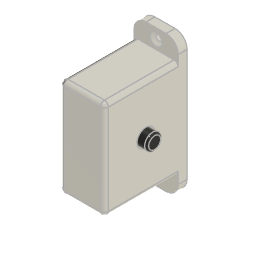
Exit Button Holder v2 (Autodesk Fusion 360 design; units mm, degrees)
Autodesk Fusion 360 part; units mm, degrees
note: some values were not read from the file. Set by a fixed rule: which sketch regions a step uses.
sketch "Sketch2" plane through (0, 0, 0) normal (1, 0, 0) x (0, 1, 0) in component "Switch PCB"
  line L0 (-3, 0) -> (-26, 0)
  line L1 (-29, 3) -> (-29, 33.5)
  line L2 (-26, 36.5) -> (-3, 36.5)
  line L3 (0, 33.5) -> (0, 3)
  line L4 (-14.5, 0) -> (-14.5, 3) construction
  line L5 (0, 18.25) -> (-3, 18.25) construction
  line L6 (-3, 33.5) -> (-26, 33.5) construction
  line L7 (-26, 33.5) -> (-26, 3) construction
  line L8 (-26, 3) -> (-3, 3) construction
  line L9 (-3, 3) -> (-3, 33.5) construction
  circle A0 centre (-26, 33.5) radius 1.5
  circle A1 centre (-3, 33.5) radius 1.5
  circle A2 centre (-26, 3) radius 1.5
  circle A3 centre (-3, 3) radius 1.5
  arc A4 (-26, 36.5) -> (-29, 33.5) centre (-26, 33.5) ccw
  arc A5 (0, 33.5) -> (-3, 36.5) centre (-3, 33.5) ccw
  arc A6 (-29, 3) -> (-26, 0) centre (-26, 3) ccw
  arc A7 (-3, 0) -> (0, 3) centre (-3, 3) ccw
  line L10 (-8.65, 7.5) -> (-20.35, 7.5)
  line L11 (-20.35, 7.5) -> (-20.35, 0)
  line L12 (-20.35, 0) -> (-8.65, 0)
  line L13 (-8.65, 0) -> (-8.65, 7.5)
  line L14 (-14.5, 0) -> (-14.5, 18.25) construction
  line L15 (-14.5, 18.25) -> (0, 18.25) construction
  circle A8 centre (-14.5, 18.25) radius 4
  circle A9 centre (-14.5, 18.25) radius 5.5
  line L16 (-6.15, 7.5) -> (-22.85, 7.5)
  line L17 (-22.85, 7.5) -> (-22.85, 0)
  line L18 (-22.85, 0) -> (-6.15, 0)
  line L19 (-6.15, 0) -> (-6.15, 7.5)
  point P0 (-29, 0)
  point P1 (0, 36.5)
  point P2 (-14.5, 3)
  point P3 (-3, 18.25)
  point P4 (-14.5, 0)
  point P5 (-14.5, -4)
  point P6 (-14.5, 0)
  dimension "d11" = 29
  dimension "d12" = 36.5
  dimension "d13" = 3
  dimension "d14" = 3
  dimension "d15" = 3
  dimension "d16" = 3
  dimension "d17" = 3
  dimension "d18" = 3
  dimension "d19" = 3
  dimension "d20" = 3
  dimension "d21" = 3
  dimension "d22" = 3
  dimension "d23" = 23
  dimension "d24" = 30.5
  dimension "d25" = 11.7
  dimension "d26" = 7.5
  dimension "d27" = 4
  dimension "d164" = 8
  dimension "d165" = 11
  dimension "d175" = 16.7
  dimension "d176" = 7.5
  constraint horizontal L0
  constraint vertical L1
  constraint horizontal L2
  constraint vertical L3
  constraint perpendicular L0 L4
  constraint perpendicular L3 L5
  constraint horizontal L6
  constraint vertical L7
  constraint horizontal L8
  constraint vertical L9
  constraint midpoint L8 P2
  constraint coincident P2 L4.end
  constraint midpoint L9 P3
  constraint coincident P3 L5.end
  constraint coincident L6.end L7.start
  constraint coincident L6.start L9.end
  constraint coincident L7.end L8.start
  constraint coincident L8.end L9.start
  constraint tangent L1 A4
  constraint tangent L2 A4
  constraint coincident L3 L5.start
  constraint coincident P1 L2
  constraint coincident P1 L3
  constraint tangent L2 A5
  constraint tangent L3 A5
  constraint coincident L0 P6
  constraint coincident P0 L1
  constraint coincident P0 L0
  constraint tangent L1 A6
  constraint tangent L0 A6
  constraint coincident origin L3
  constraint coincident origin L0
  constraint tangent L3 A7
  constraint tangent L0 A7
  constraint horizontal L10
  constraint vertical L11
  constraint horizontal L12
  constraint vertical L13
  constraint midpoint L12 P6
  constraint coincident P6 L4.start
  constraint coincident P6 P4
  constraint vertical L14
  constraint horizontal L15
  constraint coincident L14.end L15.start
  constraint horizontal L16
  constraint vertical L17
  constraint horizontal L18
  constraint vertical L19
  constraint midpoint L18 P6
  measures "d11" distance of origin P0
  measures "d12" distance of origin P1
  measures "d13" distance of P6 P2
  measures "d14" distance of L5.start P3
  measures "d15" diameter of A0
  measures "d16" diameter of A1
  measures "d17" diameter of A2
  measures "d18" diameter of A3
  measures "d19" radius of A4
  measures "d20" radius of A5
  measures "d21" radius of A6
  measures "d22" radius of A7
  measures "d23" distance of L7.end L8.end
  measures "d24" distance of L6.end L7.end
  measures "d25" distance of L10.start L10.end
  measures "d26" distance of L10.start L12.end
  measures "d27" distance of P6 P5
  measures "d164" diameter of A8
  measures "d165" diameter of A9
  measures "d175" distance of L16.start L16.end
  measures "d176" distance of L16.start L18.end
extrude "Extrude1" add sketch "Sketch2" against normal blind 1.6 contours L0 L1 L2 L3 A4 A5 A6 A7 L10 L16 L17 L19 | L0 L13 L16 L18 L19 | L0 L10 L11 L12 L13 L16 L18 | L0 L11 L16 L17 L18 | A8 | A9 makes body 1 in component "Switch PCB"
extrude "Extrude2" add sketch "Sketch2" along normal blind 5 contours L0 L10 L11 L12 L13 L16 L18 bodies 1 in component "Switch PCB"
extrude "Extrude3" add sketch "Sketch2" against normal blind 5 from surface at -1.6 contours L0 L13 L16 L18 L19 | L0 L10 L11 L12 L13 L16 L18 | L0 L11 L16 L17 L18 bodies 1 in component "Switch PCB"
sketch "Sketch1" plane through (0, 0, 0) normal (0, 1, 0) x (1, 0, 0) in component "PIR Holder"
  line L0 (0, 0) -> (0, -5) construction
  circle A0 centre (0, -5) radius 1.5
  line L1 (-11, -68) -> (11, -68)
  line L2 (11, -68) -> (11, 0)
  line L3 (11, 0) -> (-11, 0)
  line L4 (-11, 0) -> (-11, -68)
  line L5 (0, -68) -> (0, -63) construction
  circle A1 centre (0, -63) radius 1.5
  dimension "d1" = 5
  dimension "d2" = 3
  dimension "d3" = 22
  dimension "d4" = 68
  dimension "d5" = 5
  dimension "d6" = 3
  constraint coincident L0.start origin
  constraint vertical L0
  constraint coincident L0.end A0.centre
  constraint horizontal L1
  constraint vertical L2
  constraint horizontal L3
  constraint vertical L4
  constraint midpoint L3 L0.start
  constraint midpoint L1 L5.start
  constraint perpendicular L1 L5
  constraint coincident L5.end A1.centre
  measures "d1" distance of L0.start L0.end
  measures "d2" diameter of A0
  measures "d3" distance of L1.start L1.end
  measures "d4" distance of L1.start L3.end
  measures "d5" distance of L5.start L5.end
  measures "d6" diameter of A1
extrude "Extrude1'" add sketch "Sketch1" against normal blind 4.5 separate body makes body 2 in component "PIR Holder"
fillet "Fillet1" radius 6 4 edges at (11, -2.25, 68) (-11, -2.25, 68) (11, -2.25, 0) (-11, -2.25, 0) on bodies 2 in component "PIR Holder"
sketch "Sketch2 (2)" plane through (-11, 0, 0) normal (-1, 0, 0) x (0, -1, 0) in component "PIR Holder"
  line L0 (0, 6) -> (4.5, 6)
  line L1 (4.5, 6) -> (4.5, 62)
  line L2 (4.5, 62) -> (0, 62)
  line L3 (0, 62) -> (0, 6)
  line L4 (4.5, 62) -> (4.5, 6)
  line L5 (0, 0) -> (0, 15) construction
  line L6 (0, 15) -> (9, 15) construction
  dimension "d64" = 15
  dimension "d65" = 9
  constraint coincident L5.start origin
  constraint parallel L3 L5
  constraint perpendicular L4 L6
  measures "d64" distance of L5.start L5.end
  measures "d65" distance of L5.end L6.end
sketch "Sketch3" plane through (0, 0, 0) normal (1, 0, 0) x (0, 1, 0) in component "PIR Holder"
  line L0 (-32, 52.5) -> (-9, 52.5)
sketch "Sketch4" plane through (11, 0, 0) normal (1, 0, 0) x (0, 1, 0) in component "PIR Holder"
  line L0 (-4.5, 6) -> (0, 6)
  line L1 (0, 6) -> (0, 62)
  line L2 (0, 62) -> (-4.5, 62)
  line L3 (-4.5, 62) -> (-4.5, 6)
  line L4 (-26.35, 16) -> (-26.35, 23.5)
  line L5 (-26.35, 23.5) -> (-14.65, 23.5)
  line L6 (-14.65, 23.5) -> (-14.65, 16)
  line L7 (-14.65, 16) -> (-9, 16)
  arc A0 (-9, 16) -> (-6, 19) centre (-9, 19) ccw
  line L8 (-6, 19) -> (-6, 49.5)
  arc A1 (-6, 49.5) -> (-9, 52.5) centre (-9, 49.5) ccw
  line L9 (-9, 52.5) -> (-32, 52.5)
  arc A2 (-32, 52.5) -> (-35, 49.5) centre (-32, 49.5) ccw
  line L10 (-35, 49.5) -> (-35, 19)
  arc A3 (-35, 19) -> (-32, 16) centre (-32, 19) ccw
  line L11 (-32, 16) -> (-26.35, 16)
  circle A4 centre (-32, 19) radius 1.5
  circle A5 centre (-9, 49.5) radius 1.5
  circle A6 centre (-9, 19) radius 1.5
  circle A7 centre (-32, 49.5) radius 1.5
  line L12 (-14.65, 16) -> (-14.65, 23.5)
  line L13 (-14.65, 23.5) -> (-26.35, 23.5)
  line L14 (-26.35, 23.5) -> (-26.35, 16)
  line L15 (-26.35, 16) -> (-14.65, 16)
  line L16 (-20.5, 52.5) -> (-20.5, 56.5) construction
  line L17 (-20.5, 56.5) -> (-4.5, 56.5)
  line L18 (-4.5, 56.5) -> (-4.5, 12)
  line L19 (-20.5, 56.5) -> (-32, 56.5)
  line L20 (-32, 56.5) -> (-39, 56.5)
  line L21 (-39, 56.5) -> (-39, 12)
  line L22 (-39, 12) -> (-4.5, 12)
  circle A8 centre (-32, 49.5) radius 3
  circle A9 centre (-9, 49.5) radius 3
  circle A10 centre (-32, 19) radius 3
  circle A11 centre (-9, 19) radius 3
  circle A12 centre (-32, 49.5) radius 1
  circle A13 centre (-9, 49.5) radius 1
  circle A14 centre (-32, 19) radius 1
  circle A15 centre (-9, 19) radius 1
  line L23 (-35, 34.25) -> (-39, 34.25) construction
  line L24 (-32, 52.5) -> (-32, 56.5) construction
  line L25 (-20.5, 16) -> (-20.5, 12) construction
  circle A16 centre (-20.5, 34.25) radius 4
  circle A17 centre (-20.5, 34.25) radius 4.5
  point P0 (-20.5, 52.5)
  dimension "d82" = 4
  dimension "d89" = 6
  dimension "d90" = 6
  dimension "d91" = 6
  dimension "d92" = 6
  dimension "d93" = 2
  dimension "d94" = 2
  dimension "d95" = 2
  dimension "d96" = 2
  dimension "d163" = 4
  dimension "d178" = 4
  dimension "d179" = 0.5
  constraint coincident L3 L18.end
  constraint coincident L3 L17.end
  constraint perpendicular L3 L17
  constraint perpendicular L16 L19
  constraint perpendicular L16 L20
  constraint concentric A2 A8
  constraint concentric A1 A9
  constraint concentric A3 A10
  constraint concentric A0 A11
  constraint concentric A8 A12
  constraint concentric A9 A13
  constraint concentric A10 A14
  constraint concentric A11 A15
  constraint vertical L16
  constraint midpoint L9 P0
  constraint coincident P0 L16.start
  constraint midpoint L10 L23.start
  constraint midpoint L21 L23.end
  constraint coincident L9.end A2.start
  constraint vertical L24
  constraint vertical L21
  constraint horizontal L22
  constraint midpoint L15 L25.start
  constraint coincident L22 L25.end
  constraint perpendicular L22 L25
  constraint coincident L18 L22.end
  constraint coincident L18.end L22.end
  measures "d82" distance of P0 L16.end
  measures "d89" diameter of A8
  measures "d90" diameter of A9
  measures "d91" diameter of A10
  measures "d92" diameter of A11
  measures "d93" diameter of A12
  measures "d94" diameter of A13
  measures "d95" diameter of A14
  measures "d96" diameter of A15
  measures "d163" distance of L23.start L23.end
  measures "d178" distance of L25.start L25.end
extrude "Extrude5" add sketch "Sketch2" along normal blind 7.3 contours A8 | A9 bodies 1 in component "Switch PCB"
extrude "Extrude6" add sketch "Sketch2" along normal blind 6.8 from surface at 7.3 contours A8 bodies 1 in component "Switch PCB"
fillet "Fillet1'" radius 1 1 edges at (14.1, -18.2293, 16.8035) on bodies 1 in component "Switch PCB"
fillet "Fillet2" radius 1 1 edges at (7.3, -19.6278, 16.2611) on bodies 1 in component "Switch PCB"
chamfer "Chamfer1" distance 1 angle 45 4 edges at (5, -20.35, 3.75) (5, -8.65, 3.75) (-6.6, -22.85, 3.75) (-6.6, -6.15, 3.75) on bodies 1 in component "Switch PCB"
extrude "Extrude2'" add sketch "Sketch4" against normal blind 2 contours L3 L17 L18 L19 L20 L21 L22 | L4 L5 L6 L7 L8 L9 L10 L11 L12 L13 L14 A8 A9 A10 A11 | L4 L5 L6 L12 L13 L14 L15 | A3 A10 | A0 A11 | A2 A8 | A1 A9 | A4 | A5 | A6 | A7 | A12 | A13 | A14 | A15 bodies 2 in component "PIR Holder"
extrude "Extrude4" add sketch "Sketch4" against normal up to surface (7.75 mm away) from surface at -2 contours A3 A10 | A0 A11 | A2 A8 | A1 A9 | A4 | A5 | A6 | A7 bodies 2 in component "PIR Holder"
sketch "Sketch5" plane through (11, 0, 0) normal (1, 0, 0) x (0, 1, 0) in component "PIR Holder"
  line L0 (-20.5, 56.5) -> (-32, 56.5)
  line L1 (-20.5, 56.5) -> (-4.5, 56.5)
  line L2 (-32, 56.5) -> (-39, 56.5)
  line L3 (-39, 56.5) -> (-39, 12)
  line L4 (-39, 12) -> (-4.5, 12)
  line L5 (-4.5, 56.7) -> (-4.5, 56.5)
  line L6 (-4.5, 12.2) -> (-4.5, 10)
  line L7 (-4.5, 56.7) -> (-4.5, 12.2) construction
  line L8 (-7.5, 51.2) -> (-4.5, 51.2)
  line L9 (-4.5, 51.2) -> (-4.5, 56.7)
  line L10 (-41.2, 9.8) -> (-4.5, 9.8)
  line L11 (-41.2, 58.7) -> (-41.2, 9.8)
  line L12 (-4.5, 12) -> (-4.5, 9.8)
  line L13 (-41.2, 58.7) -> (-4.5, 58.7)
  line L14 (-4.5, 58.7) -> (-4.5, 12)
  line L15 (-20.5, 56.5) -> (-20.5, 58.7) construction
  dimension "d180" = 2.2
  constraint coincident L1.end L5.end
  constraint perpendicular L1 L5
  constraint coincident L7 L8.end
  constraint perpendicular L7 L8
  constraint coincident L4.end L12.start
  constraint perpendicular L10 L12
  constraint perpendicular L5 L13
  constraint perpendicular L4 L14
  constraint coincident L0.start L1.start
  constraint coincident L13 L15.end
  constraint perpendicular L13 L15
  measures "d180" distance of L0.start L15.end
extrude "Extrude5'" add sketch "Sketch5" against normal up to surface (20 mm away) contours L0 L1 L2 L3 L4 L5 L6 L9 L10 L11 L12 L13 L14 bodies 2 in component "PIR Holder"
sketch "Sketch6" plane through (0, 0, 12) normal (0, 0, 1) x (1, 0, 0) in component "PIR Holder"
  line L0 (-9, -39) -> (9, -39)
  line L1 (-9, -4.5) -> (-9, -39)
  line L2 (9, -4.5) -> (-9, -4.5)
  line L3 (6.25, -15.65) -> (6.25, -25.35)
  line L4 (1.25, -14.65) -> (5.25, -14.65)
  line L5 (1.25, -26.35) -> (5.25, -26.35)
  line L6 (0.75, -42.3) -> (9.25, -42.3)
  line L7 (9, -39) -> (9, -4.5)
  line L8 (-5.35, -13.15) -> (-4.35, -12.15)
  line L9 (-4.35, -12.15) -> (-0.35, -12.15)
  line L10 (-0.35, -12.15) -> (-0.35, -9)
  line L11 (-0.35, -9) -> (1.25, -9)
  line L12 (1.25, -9) -> (1.25, -14.65)
  line L13 (1.25, -14.65) -> (5.25, -14.65)
  line L14 (5.25, -14.65) -> (6.25, -15.65)
  line L15 (6.25, -15.65) -> (6.25, -25.35)
  line L16 (6.25, -25.35) -> (5.25, -26.35)
  line L17 (5.25, -26.35) -> (1.25, -26.35)
  line L18 (1.25, -26.35) -> (1.25, -32)
  line L19 (1.25, -32) -> (-0.35, -32)
  line L20 (-0.35, -32) -> (-0.35, -28.85)
  line L21 (-0.35, -28.85) -> (-4.35, -28.85)
  line L22 (-4.35, -28.85) -> (-5.35, -27.85)
  line L23 (-5.35, -27.85) -> (-5.35, -13.15)
  line L24 (-0.35, -12.15) -> (1.25, -14.65)
  line L25 (-0.35, -28.85) -> (1.25, -26.35)
  constraint coincident L9.end L10.start
  constraint coincident L4.start L12.end
  constraint coincident L20.end L21.start
  constraint coincident L5.start L17.end
extrude "Extrude6'" cut sketch "Sketch6" against normal up to surface (2.2 mm away) contours L3 L4 L5 L8 L9 L13 L14 L15 L16 L17 L21 L22 L23 L24 L25 bodies 2 in component "PIR Holder"
chamfer "Chamfer3" distance 1.5 angle 45 2 edges at (-1.3985, -4.5, 63.5424) (-1.3985, -4.5, 5.5424) on bodies 2 in component "PIR Holder"
sketch "Sketch1 (2)" plane through (-9, 0, 0) normal (-1, 0, 0) x (0, -1, 0) in component "PIR Holder Lid"
  line L0 (39, 12) -> (4.5, 12)
  line L1 (39, 56.5) -> (39, 12)
  line L2 (4.5, 56.5) -> (39, 56.5)
  line L3 (41.2, 9.8) -> (41.2, 58.7)
  line L4 (4.5, 9.8) -> (41.2, 9.8)
  line L5 (4.5, 9.8) -> (41.2, 9.8)
  line L6 (4.5, 58.7) -> (4.5, 56.5)
  line L7 (39, 12) -> (4.5, 12)
  circle A0 centre (32, 19) radius 1.5
  circle A1 centre (32, 19) radius 1
  line L8 (41.2, 9.8) -> (4.5, 9.8) construction
  line L9 (4.5, 9.8) -> (5, 9.8) construction
  line L10 (4.5, 58.7) -> (4.5, 56.5)
  line L11 (41.2, 9.8) -> (41.2, 58.7)
  line L12 (4.5, 56.5) -> (39, 56.5)
  line L13 (39, 56.5) -> (39, 12)
  line L14 (13.15, 23.5) -> (13.15, 16)
  line L15 (13.15, 16) -> (27.85, 16)
  line L16 (27.85, 16) -> (27.85, 23.5)
  line L17 (27.85, 23.5) -> (13.15, 23.5)
  line L18 (4.5, 12) -> (4.5, 9.8)
  line L19 (4.5, 12) -> (4.5, 9.8)
  line L20 (4.5, 58.7) -> (41.2, 58.7)
  line L21 (41.2, 58.7) -> (41.2, 9.8)
  line L22 (41.2, 9.8) -> (4.5, 9.8)
  line L23 (4.5, 9.8) -> (4.5, 58.7)
  line L24 (4.5, 56.5) -> (39, 56.5)
  line L25 (39, 56.5) -> (39, 12)
  line L26 (39, 12) -> (4.5, 12)
  line L27 (4.5, 12) -> (4.5, 56.5)
  circle A2 centre (9, 49.5) radius 1
  line L28 (41.2, 58.7) -> (4.5, 58.7)
  line L29 (41.2, 58.7) -> (4.5, 58.7)
  point P0 (32, 19)
  dimension "d124" = 2
  constraint concentric A0 A1
  constraint coincident L3.start L4.end
  constraint coincident L4.start L5.start
  constraint coincident L5 L9.end
  constraint horizontal L20
  constraint vertical L21
  constraint horizontal L22
  constraint vertical L23
  constraint horizontal L24
  constraint vertical L25
  constraint horizontal L26
  constraint vertical L27
  constraint coincident L0.start L1.end
  constraint coincident L2.start L6.end
  constraint collinear L20 L28
  measures "d124" diameter of A1
extrude "Extrude1''" add sketch "Sketch1 (2)" along normal up to surface (2 mm away) separate body contours L0 L1 L2 L3 L4 L5 L6 L7 L10 L11 L12 L13 L18 L19 L20 L21 L22 L23 L24 L25 L26 L28 L29 | L0 L1 L2 L7 L12 L13 L23 L24 L25 L26 L27 | A0 | L14 L15 L16 L17 makes body 3 in component "PIR Holder Lid"
extrude "Extrude2''" add sketch "Sketch1 (2)" against normal blind 2 contours L0 L1 L2 L7 L12 L13 L23 L24 L25 L26 L27 | A0 | L14 L15 L16 L17 bodies 3 in component "PIR Holder Lid"
chamfer "Chamfer2" distance 1.6 angle 45 2 edges at (-11, -8.0677, 49.1384) (-11, -31.0677, 18.6384) on bodies 3 in component "PIR Holder Lid"
fillet "Fillet4" radius 2 2 edges at (-10, -41.2, 9.8) (-10, -41.2, 58.7) on bodies 3 in component "PIR Holder Lid"
fillet "Fillet5" radius 2 5 edges at (-11, -21.85, 58.7) (-11, -40.6142, 58.1142) (-11, -41.2, 34.25) (-11, -40.6142, 10.3858) (-11, -21.85, 9.8) on bodies 3 in component "PIR Holder Lid"
fillet "Fillet4'" radius 2 2 edges at (1, -41.2, 9.8) (1, -41.2, 58.7) on bodies 2 in component "PIR Holder"
fillet "Fillet5'" radius 2 5 edges at (11, -21.85, 58.7) (11, -40.6142, 58.1142) (11, -41.2, 34.25) (11, -40.6142, 10.3858) (11, -21.85, 9.8) on bodies 2 in component "PIR Holder"
component "Switch PCB" placed x (1, 0, 0) y (0, 1, 0) z (0, 0, 1) at (1.25, -6, 16)
component "PIR Holder" placed x (1, 0, 0) y (0, 1, 0) z (0, 0, 1) at (0, 0, 0)
component "PIR Holder Lid" placed x (1, 0, 0) y (0, 1, 0) z (0, 0, 1) at (0, 0, 0)
named bodies: "Button Holder", "Button Holder Lid"
